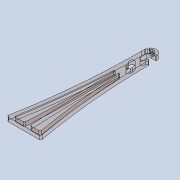
# Autodesk Inventor part: wing
Saved by Autodesk Inventor 2020 (Build 240168000, 168)
## iProperties
Created: 2021-02-23
Part Number: wing
Material: ポリカーボネート、スモーク
Document SubType Name: Modeling
Designer: AA19065
Density: 1.2 g/cm^3
Appearance: ポリカーボネート - スモーク
Author: AA19065
Autodesk Inventor part; units mm, degrees
ref_plane "YZ Plane" through (0, 0, 0) normal (1, 0, 0) x (0, 1, 0)
ref_plane "XZ Plane" through (0, 0, 0) normal (0, 1, 0) x (-1, 0, 0)
ref_plane "XY Plane" through (0, 0, 0) normal (0, 0, 1) x (1, 0, 0)
sketch "スケッチ1" plane through (0, 0, 0) normal (0, 1, 0) x (-1, 0, 0)
  circle A0 centre (0, 0) radius 3 construction
  circle A1 centre (0, 21.2) radius 3 construction
  line L0 (3, 24.2) -> (-3, 24.2) construction
  line L1 (-3, 24.2) -> (-3, -3) construction
  line L2 (-3, -3) -> (3, -3) construction
  line L3 (3, -3) -> (3, 24.2) construction
  circle A2 centre (0, 21.2) radius 3.5
  circle A3 centre (0, 0) radius 3.5 construction
  line L4 (0, 21.2) -> (-4, 25.2)
  line L5 (-4, 25.2) -> (-4, 30.2)
  circle A4 centre (-4, 30.2) radius 3.5
  line L6 (-0.5, 30.2) -> (-0.5, 26.6497)
  line L7 (-0.5, 26.6497) -> (2.4749, 23.6749)
  line L8 (-7.5, 30.2) -> (-7.5, 23.7503)
  line L9 (-7.5, 23.7503) -> (-2.4749, 18.7251)
  arc A5 (-0.5, 28.3066) -> (0.6716, 25.4782) centre (3.5, 28.3066) ccw
  arc A6 (-7.5, 28.3066) -> (-4.2782, 20.5284) centre (3.5, 28.3066) ccw
  circle A7 centre (-4, 9) radius 3.5
  line L10 (2.4749, 2.4749) -> (0.6716, 4.2782) construction
  arc A8 (-0.5, 7.1066) -> (0.6716, 4.2782) centre (3.5, 7.1066) ccw construction
  line L11 (-10.5, 0.2919) -> (-10.5, -4)
  line L12 (6.5, -4) -> (6.5, 0.2919)
  arc A9 (-10.5, -4) -> (6.5, -4) centre (-2, -4) ccw
  arc A10 (23, 181.2) -> (6.5, 0.2919) centre (1006.5, 0.2919) ccw
  arc A11 (-10.5, 0.2919) -> (-27, 181.2) centre (-1010.5, 0.2919) ccw
  line L13 (6.124, -6.5) -> (-3, -6.5)
  line L14 (-3, -6.5) -> (-3, -9.5)
  line L15 (-3, -9.5) -> (6.124, -9.5)
  line L16 (6.124, -9.5) -> (6.124, -6.5)
  arc A12 (4.4807, -9.5) -> (2.9559, -9.5) centre (3.7183, -8.8529) ccw
  arc A13 (1.0407, -9.5) -> (2.8258, -8.402) centre (1.0407, -7.5) ccw
  line L17 (23, 181.2) -> (-27, 181.2)
  circle A14 centre (-4, 0) radius 3.5
  line L18 (-0.5, 9) -> (-0.5, 0)
  line L19 (-7.5, 0) -> (-7.5, 9)
  line L20 (-4, 3.5) -> (-10.5, 3.5)
  line L21 (-10.5, 3.5) -> (-10.5, -3.5)
  line L22 (-10.5, -3.5) -> (-4, -3.5)
  line L23 (-4, -3.5) -> (-4, 3.5) construction
  arc A15 (-10.5, 6) -> (-7.5, 9) centre (-10.5, 9) ccw
  line L24 (-10.5, 6) -> (-10.6533, 6)
  point P0 (0, -3)
  point P1 (-3, -8)
  point P2 (-10.5, 0)
  point P3 (-7.5, 3.5)
  point P4 (-10.5163, 6)
  dimension "d7" = 7
  dimension "d0" = 6
  dimension "d1" = 6
  dimension "d2" = 21.2
  dimension "d3" = 27.2
  dimension "d4" = 3
  dimension "d5" = 6
  dimension "d6" = 7
  dimension "d8" = 5
  dimension "d9" = 135
  dimension "d10" = 4
  dimension "d11" = 4
  dimension "d12" = 21.2
  dimension "d14" = 6.5
  dimension "d15" = 4
  dimension "d17" = 3
  dimension "d18" = 1
  dimension "d19" = 2
  dimension "d20" = 1000
  dimension "d21" = 50
  dimension "d22" = 160
  dimension "d23" = 3
  dimension "d24" = 6.5
  dimension "d25" = 2.5
  constraints: 50 end point, 30 point on circle, 19 tangent, 15 centre point, 11 point on line, 8 parallel, 5 coincident, 5 horizontal, 4 equal radius, 4 horizontal alignment, 4 midpoint, 4 vertical alignment, 3 perpendicular, 1 concentric, 1 line through centre, 1 vertical, 7 other
  measures "d0" diameter of A0
  measures "d1" diameter of A1
  measures "d2" distance of A0.centre A1.centre
  measures "d3" distance of L0.end L1.end
  measures "d4" distance from line of L2 point (0, 0)
  measures "d5" distance of L1.end L2.end
  measures "d6" diameter of A2
  measures "d8" distance of L4.end L5.end
  measures "d9" angle of L5 L4
  measures "d10" distance from line of A1.centre L5
  measures "d11" radius of A5
  measures "d12" distance of A4.centre A7.centre
  measures "d14" distance from line of L12 L4.start
  measures "d15" vertical distance of point (0, 0) L12.start
  measures "d17" distance of L13.end L14.end
  measures "d18" radius of A12
  measures "d19" radius of A13
  measures "d20" radius of A10
  measures "d21" distance of L17.end L17.start
  measures "d22" distance from line of A1.centre L17
  measures "d23" distance between parallel lines of L11 L8
  measures "d24" distance from line of L13 point (0, 0)
  measures "d25" distance from line of L20 L24.start
extrude "押し出し1" add sketch "スケッチ1" along normal blind 6 contours L9 L8 A6 | A7 A15 L24 A11 L17 A10 L12 A9 L13 L14 L15 L11 L22 A14 L18 | L15 A12 | L15 A13 A12
fillet "フィレット1" radius 1 5 edges at (10.5163, 3, 6) (3, 3, -9.5) (3, 3, -6.5) (-6.124, 3, -6.5) (10.5, 3, -3.5)
sketch "スケッチ2" plane through (0, 6, 0) normal (0, 1, 0) x (1, 0, 0)
  arc A0 (9.4833, 3.5) -> (10.4811, 4.5667) centre (9.4833, 4.5) ccw projected
  arc A1 (10.4811, 4.5667) -> (-4.4807, 9.5) centre (2, 4) ccw projected
  arc A2 (-4.4807, 9.5) -> (-2.8258, 8.402) centre (-3.7183, 8.8529) ccw projected
  arc A3 (-1.0407, 9.5) -> (-2.8258, 8.402) centre (-1.0407, 7.5) ccw projected
  line L0 (-1.0407, 9.5) -> (2, 9.5) projected
  arc A4 (3, 8.5) -> (2, 9.5) centre (2, 8.5) ccw projected
  line L1 (3, 8.5) -> (3, 7.5) projected
  arc A5 (2, 6.5) -> (3, 7.5) centre (2, 7.5) ccw projected
  line L2 (2, 6.5) -> (-5.3485, 6.5) projected
  arc A6 (-5.3485, 6.5) -> (-6.3283, 5.7) centre (-5.3485, 5.5) ccw projected
  arc A7 (-6.3283, 5.7) -> (-6.5, 4) centre (2, 4) ccw projected
  line L3 (-6.5, 4) -> (-6.5, -0.2919) projected
  arc A8 (-23, -181.2) -> (-6.5, -0.2919) centre (-1006.5, -0.2919) ccw projected
  line L4 (-23, -181.2) -> (27, -181.2) projected
  arc A9 (10.5242, -7.2472) -> (27, -181.2) centre (1010.5, -0.2919) ccw projected
  arc A10 (10.5242, -7.2472) -> (9.0363, -6.3813) centre (9.5242, -7.2542) ccw projected
  arc A11 (9.0363, -6.3813) -> (7.5, -9) centre (10.5, -9) ccw projected
  arc A12 (0.5, -9) -> (7.5, -9) centre (4, -9) ccw projected
  line L5 (0.5, -9) -> (0.5, 0) projected
  arc A13 (4, 3.5) -> (0.5, 0) centre (4, 0) ccw projected
  line L6 (4, 3.5) -> (9.4833, 3.5) projected
  arc A14 (7.5, -28.3066) -> (4.2782, -20.5284) centre (-3.5, -28.3066) ccw projected
  line L7 (7.5, -28.3066) -> (7.5, -30.2) projected
  arc A15 (0.5, -30.2) -> (7.5, -30.2) centre (4, -30.2) ccw projected
  line L8 (0.5, -30.2) -> (0.5, -28.3066) projected
  arc A16 (0.5, -28.3066) -> (-0.6716, -25.4782) centre (-3.5, -28.3066) ccw projected
  line L9 (-0.6716, -25.4782) -> (-2.4749, -23.6749) projected
  arc A17 (2.4749, -18.7251) -> (-2.4749, -23.6749) centre (0, -21.2) ccw projected
  line L10 (2.4749, -18.7251) -> (4.2782, -20.5284) projected
  arc A18 (-17.0146, -176.2) -> (-2.5039, -45.2) centre (-1006.5, -0.2919) ccw
  arc A19 (6.5039, -45.2) -> (21.0146, -176.2) centre (1010.5, -0.2919) ccw
  arc A20 (-23, -181.2) -> (-6.5, -0.2919) centre (-1006.5, -0.2919) ccw projected
  arc A21 (10.5242, -7.2472) -> (27, -181.2) centre (1010.5, -0.2919) ccw projected
  arc A22 (-0.406, -45.2) -> (-2.5039, -45.2) centre (-1.4549, -45.2469) ccw
  arc A23 (6.5039, -45.2) -> (4.406, -45.2) centre (5.4549, -45.2469) ccw
  arc A24 (-2.0146, -176.2) -> (-0.406, -45.2) centre (-1332.9861, -94.346) ccw
  arc A25 (4.406, -45.2) -> (6.0146, -176.2) centre (1336.9861, -94.346) ccw
  line L11 (-17.0146, -176.2) -> (-2.0146, -176.2)
  line L12 (6.0146, -176.2) -> (21.0146, -176.2)
  line L13 (0.5, -9) -> (0.5, 0) projected
  point P0 (0, 0)
  dimension "d38" = 15
  dimension "d39" = 5
  dimension "d40" = 5
  dimension "d41" = 1.05
  dimension "d42" = 1.05
  dimension "d43" = 15
  dimension "d44" = 15
  dimension "d46" = 5
  constraints: 12 point on circle, 6 centre point, 6 horizontal alignment, 4 end point, 3 tangent, 2 concentric, 2 horizontal, 1 equal radius
  measures "d38" vertical distance of A15.centre A18.end
  measures "d39" radial gap between concentric circles of A8 A18
  measures "d40" radial gap between concentric circles of A9 A19
  measures "d41" radius of A23
  measures "d42" radius of A22
  measures "d43" distance of L11.end L11.start
  measures "d44" distance of L12.end L12.start
  measures "d46" distance from line of L4 L11.end
extrude "押し出し3" cut sketch "スケッチ2" against normal blind 5.7 contours A18 A22 A24 L11 | A19 L12 A25 A23
fillet "フィレット2" radius 2 6 edges at (-17.0146, 3.15, 176.2) (-2.0146, 3.15, 176.2) (6.0146, 3.15, 176.2) (21.0146, 3.15, 176.2) (27, 3, 181.2) (-23, 3, 181.2)
equation "\"d7\" = d6"
equation "\"d12\" = d2"
